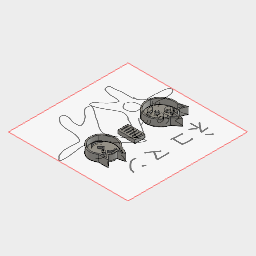
nekoman (Autodesk Fusion 360 design; units mm, degrees)
Autodesk Fusion 360 part; units mm, degrees
sketch "スケッチ1" plane through (0, 0, 0) normal (0, 1, 0) x (1, 0, 0)
  arc A0 (10.5126, 63.76) -> (-16.5243, 47.5379) centre (5.362, 41.7026) ccw
  line L0 (10.5126, 63.76) -> (21.654, 66.602)
  line L1 (21.654, 66.602) -> (18.1432, 56.8499)
  line L2 (18.1432, 56.8499) -> (19.8986, 52.5589)
  line L3 (19.8986, 52.5589) -> (19.8986, 49.4382)
  line L4 (19.8986, 49.4382) -> (32.9665, 47.4878)
  line L5 (32.9665, 47.4878) -> (23.0193, 39.296)
  arc A1 (-7.7975, 26.0331) -> (23.0193, 39.296) centre (2.2405, 45.1429) ccw
  arc A2 (-16.5243, 47.5379) -> (-7.7975, 26.0331) centre (5.1534, 43.8117) ccw
extrude "押し出し1" add sketch "スケッチ1" along normal blind 10 makes body 1
shell "シェル1" thickness 2 removed faces 1 at (3.5389, 10, -35.3077) on bodies 1
sketch "スケッチ2" plane through (0, 2, 0) normal (0, 1, 0) x (-1, 0, 0)
  arc A0 (-10.522, -61.6984) -> (14.5683, -47.11) centre (-5.362, -41.7026) ccw
  arc A1 (14.5683, -47.11) -> (6.7378, -27.7362) centre (-5.1534, -43.8117) ccw
  arc A2 (6.7378, -27.7362) -> (-21.2509, -40.4306) centre (-2.2405, -45.1429) ccw
  line L0 (-21.2509, -40.4306) -> (-28.2244, -46.1734)
  line L1 (-28.2244, -46.1734) -> (-17.8986, -47.7146)
  line L2 (-17.8986, -47.7146) -> (-17.8986, -52.1657)
  line L3 (-17.8986, -52.1657) -> (-16.0011, -56.8041)
  line L4 (-16.0011, -56.8041) -> (-18.4952, -63.7322)
  line L5 (-18.4952, -63.7322) -> (-10.522, -61.6984)
  arc A3 (-12.2642, -52.0039) -> (-6.2082, -61.1255) centre (0.1091, -50.3601) ccw
  arc A4 (-10.2897, -51.7286) -> (-5, -60) centre (-3.653, -53.3114) ccw
  line L6 (-10.2897, -51.7286) -> (-12.2642, -52.0039)
  line L7 (-5, -60) -> (-6.2082, -61.1255)
  arc A5 (-17.3568, -38.653) -> (-12.2642, -46.9113) centre (-9.4779, -39.4937) ccw
  arc A6 (-16.2223, -39.4937) -> (-12.2642, -45.5349) centre (-8.9959, -39.0763) ccw
  line L8 (-16.2223, -39.4937) -> (-17.3568, -38.653)
  line L9 (-12.2642, -45.5349) -> (-12.2642, -46.9113)
  ellipse E0 centre (-3.653, -54.619) end of major axis (-5.2447, -50.3601) minor radius 2.952
  line L10 (-2.0613, -58.8778) -> (-5.2447, -50.3601)
  line L11 (-0.8878, -53.5855) -> (-6.4182, -55.6524)
  ellipse E1 centre (-7.8598, -39.4937) end of major axis (-11.0255, -34.1109) minor radius 3.1255
  line L12 (-4.6941, -44.8764) -> (-11.0255, -34.1109)
  line L13 (-5.1657, -37.9092) -> (-10.5539, -41.0781)
  arc A7 (3, -42) -> (-0.7318, -45.1429) centre (0.8115, -43.1885) ccw
  arc A8 (3, -43.1885) -> (0.8115, -45.1429) centre (1.3751, -43.5714) ccw
  line L14 (-0.7318, -45.1429) -> (0.8115, -45.1429)
  line L15 (3, -43.1885) -> (3, -42)
  ellipse E2 centre (8, -40) end of major axis (5.654, -35.1095) minor radius 2.3132
  line L16 (10.346, -44.8905) -> (5.654, -35.1095)
  line L17 (10.0856, -38.9995) -> (5.9144, -41.0005)
extrude "押し出し2" add sketch "スケッチ2" along normal blind 2 contours A3 A4 L6 L7 | A5 A6 L8 L9 | E0 L10 L11 | E0 L10 L11 | E0 L10 L11 | E0 L10 L11 | E1 L12 L13 | E1 L12 L13 | E1 L12 L13 | E1 L12 L13 | A7 A8 L14 L15 | E2 L16 L17 | E2 L16 L17 | E2 L16 L17 | E2 L16 L17 bodies 1
sketch "スケッチ3" plane through (0, 4, 0) normal (0, 1, 0) x (-1, 0, 0)
  ellipse E0 centre (-7.8598, -39.4937) end of major axis (-11.0255, -34.1109) minor radius 3.1255
  circle A0 centre (-8, -39) radius 0.6774
  circle A1 centre (-4, -53) radius 0.75
  dimension "d6" = 1.5
  measures "d6" diameter of A1
extrude "押し出し3" cut sketch "スケッチ3" against normal blind 1 contours A0 | A1 bodies 1
sketch "スケッチ4" plane through (0, 0, 0) normal (0, 1, 0) x (1, 0, 0)
  arc A0 (23, -32) -> (-9, -34) centre (7.8483, -46.573) ccw
  arc A1 (-9, -34) -> (-3, -60) centre (6.5187, -44.1111) ccw
  arc A2 (-3, -60) -> (17, -60) centre (7, -46.3333) ccw
  line L0 (23, -32) -> (36, -39)
  line L1 (36, -39) -> (26, -42)
  arc A3 (24, -52) -> (26, -42) centre (15, -45) ccw
  line L2 (24, -52) -> (31, -60)
  line L3 (31, -60) -> (17, -60)
extrude "押し出し4" add sketch "スケッチ4" along normal blind 10 separate body makes body 2
shell "シェル2" thickness 2 removed faces 1 at (4.87, 10, 48.9453) on bodies 2
sketch "スケッチ5" plane through (0, 2, 0) normal (0, 1, 0) x (-1, 0, 0)
  arc A0 (-21.3133, 51.9667) -> (-23.3624, 40.7032) centre (-15, 45) ccw
  line L0 (-23.3624, 40.7032) -> (-30.8005, 38.4718)
  line L1 (-30.8005, 38.4718) -> (-21.7687, 33.6085)
  arc A1 (-21.7687, 33.6085) -> (7.3588, 35.145) centre (-7.8483, 46.573) ccw
  arc A2 (7.3588, 35.145) -> (1.8929, 58.3315) centre (-6.5187, 44.1111) ccw
  arc A3 (1.8929, 58.3315) -> (-16.3236, 58) centre (-7, 46.3333) ccw
  line L2 (-16.3236, 58) -> (-26.5925, 58)
  line L3 (-26.5925, 58) -> (-21.3133, 51.9667)
  arc A4 (-9, 57) -> (-13.6956, 46.6828) centre (-8.2057, 50.4113) ccw
  arc A5 (-9, 55) -> (-12, 48) centre (-9.3333, 51) ccw
  line L4 (-13.6956, 46.6828) -> (-12, 48)
  line L5 (-9, 55) -> (-9, 57)
  arc A6 (-13, 43) -> (-16, 33) centre (-10.9286, 36.9286) ccw
  arc A7 (-13, 42) -> (-15, 34) centre (-11, 37.25) ccw
  line L6 (-13, 42) -> (-13, 43)
  line L7 (-15, 34) -> (-16, 33)
  line L8 (-8, 44) -> (-5, 40)
  line L9 (-5, 40) -> (0.3333, 44)
  line L10 (0.3333, 44) -> (-0.4908, 45.0988)
  line L11 (-0.4908, 45.0988) -> (-4.6226, 42)
  line L12 (-4.6226, 42) -> (-6.5187, 44.1111)
  line L13 (-6.5187, 44.1111) -> (-8, 44)
  arc A8 (3, 35) -> (5, 48) centre (-0.9524, 42.2619) ccw
  arc A9 (4, 34) -> (6, 48) centre (-0.8244, 41.8321) ccw
  line L14 (5, 48) -> (6, 48)
  line L15 (4, 34) -> (3, 35)
extrude "押し出し5" add sketch "スケッチ5" along normal blind 2 contours A4 A5 L4 L5 | A6 A7 L6 L7 | L8 L9 L10 L11 L12 L13 | A8 A9 L14 L15 bodies 2
sketch "スケッチ6" plane through (0, 0, 0) normal (0, -1, 0) x (1, 0, 0)
  arc A0 (26, 42) -> (24, 52) centre (15, 45) ccw
  line L0 (24, 52) -> (31, 60)
  line L1 (31, 60) -> (17, 60)
  arc A1 (17, 60) -> (-3, 60) centre (7, 46.3333) ccw
  arc A2 (-3, 60) -> (-9, 34) centre (6.5187, 44.1111) ccw
  arc A3 (-9, 34) -> (23, 32) centre (7.8483, 46.573) ccw
  line L2 (23, 32) -> (36, 39)
  line L3 (36, 39) -> (26, 42)
  circle A4 centre (8, 44) radius 2.5
  point P0 (8, 44)
  dimension "d14" = 5
  measures "d14" diameter of A4
extrude "押し出し6" cut sketch "スケッチ6" against normal blind 1.5 contours A4 bodies 2
sketch "スケッチ7" plane through (0, 0, 0) normal (0, -1, 0) x (1, 0, 0)
  arc A0 (-16.5243, -47.5379) -> (10.5126, -63.76) centre (5.362, -41.7026) ccw
  line L0 (10.5126, -63.76) -> (21.654, -66.602)
  line L1 (21.654, -66.602) -> (18.1432, -56.8499)
  line L2 (18.1432, -56.8499) -> (19.8986, -52.5589)
  line L3 (19.8986, -52.5589) -> (19.8986, -49.4382)
  line L4 (19.8986, -49.4382) -> (32.9665, -47.4878)
  line L5 (32.9665, -47.4878) -> (23.0193, -39.296)
  arc A1 (23.0193, -39.296) -> (-7.7975, -26.0331) centre (2.2405, -45.1429) ccw
  arc A2 (-7.7975, -26.0331) -> (-16.5243, -47.5379) centre (5.1534, -43.8117) ccw
  circle A3 centre (2, -43) radius 2.5
  dimension "d17" = 5
  measures "d17" diameter of A3
extrude "押し出し7" cut sketch "スケッチ7" against normal blind 1.5 contours A3 bodies 1
sketch "スケッチ8" plane through (0, 0, 0) normal (0, 1, 0) x (1, 0, 0)
  line L0 (-5, -10) -> (20, -10)
  line L1 (20, -10) -> (20, 5)
  line L2 (20, 5) -> (-5, 5)
  line L3 (-5, 5) -> (-5, -10)
  dimension "d20" = 25
  dimension "d21" = 15
  measures "d20" distance of L1 L3
  measures "d21" distance of L0 L2
extrude "押し出し8" add sketch "スケッチ8" along normal blind 5 separate body makes body 3
sketch "スケッチ9" plane through (0, 5, 0) normal (0, 1, 0) x (-1, 0, 0)
  line L0 (5, -5) -> (5, 10)
  line L1 (5, 10) -> (-20, 10)
  line L2 (-20, 10) -> (-20, -5)
  line L3 (-20, -5) -> (5, -5)
  line L4 (-18, -3) -> (-17, -3)
  line L5 (-17, -3) -> (-17, 7)
  line L6 (-17, 7) -> (-18, 7)
  line L7 (-18, 7) -> (-18, -3)
  line L8 (-14, -3) -> (-13, -3)
  line L9 (-13, -3) -> (-13, 7)
  line L10 (-13, 7) -> (-14, 7)
  line L11 (-14, 7) -> (-14, -3)
  line L12 (-10, -3) -> (-9, -3)
  line L13 (-9, -3) -> (-9, 7)
  line L14 (-9, 7) -> (-10, 7)
  line L15 (-10, 7) -> (-10, -3)
  line L16 (-6, -3) -> (-5, -3)
  line L17 (-5, -3) -> (-5, 7)
  line L18 (-5, 7) -> (-6, 7)
  line L19 (-6, 7) -> (-6, -3)
  line L20 (-2, -3) -> (-1, -3)
  line L21 (-1, -3) -> (-1, 7)
  line L22 (-1, 7) -> (-2, 7)
  line L23 (-2, 7) -> (-2, -3)
  line L24 (2, -3) -> (3, -3)
  line L25 (3, -3) -> (3, 7)
  line L26 (3, 7) -> (2, 7)
  line L27 (2, 7) -> (2, -3)
extrude "押し出し9" cut sketch "スケッチ9" against normal blind 1 contours L4 L5 L6 L7 | L8 L9 L10 L11 | L12 L13 L14 L15 | L16 L17 L18 L19 | L20 L21 L22 L23 | L24 L25 L26 L27 bodies 3
